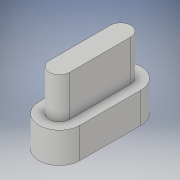
# Autodesk Inventor part: startselectButton
Saved by Autodesk Inventor 2019 (Build 230136000, 136)
## iProperties
Created: 2020-10-12
Part Number: startselectButton
Material: Generisch
Document SubType Name: Modeling
Designer: d_fel
Density: 1 g/cm^3
Appearance: Vorgabe
Author: d_fel
Autodesk Inventor part; units mm, degrees
ref_plane "YZ Plane" through (0, 0, 0) normal (1, 0, 0) x (0, 1, 0)
ref_plane "XZ Plane" through (0, 0, 0) normal (0, 1, 0) x (-1, 0, 0)
ref_plane "XY Plane" through (0, 0, 0) normal (0, 0, 1) x (1, 0, 0)
sketch "Skizze1" plane through (0, 0, 0) normal (0, 1, 0) x (-1, 0, 0)
  line L0 (4, 0) -> (4, -6)
  line L1 (0, -6) -> (0, 0)
  arc A0 (4, 0) -> (0, 0) centre (2, 0) ccw
  arc A1 (0, -6) -> (4, -6) centre (2, -6) ccw
  dimension "d0" = 4
  dimension "d1" = 6
  constraints: 4 end point, 4 point on circle, 4 tangent, 2 centre point, 1 parallel
  measures "d0" distance of L0.end L1.start
  measures "d1" distance of L0.start L0.end
extrude "Extrusion1" add sketch "Skizze1" along normal blind 3
sketch "Skizze2" plane through (0, 3, 0) normal (0, 1, 0) x (1, 0, 0)
  line L0 (-3, 0) -> (-3, 6)
  line L1 (-1, 6) -> (-1, 0)
  arc A0 (-3, 0) -> (-1, 0) centre (-2, 0) ccw
  arc A1 (-1, 6) -> (-3, 6) centre (-2, 6) ccw
  point P0 (0, 0)
  dimension "d4" = 2
  dimension "d5" = 6
  dimension "d6" = 1
  dimension "d7" = 0
  constraints: 4 end point, 4 point on circle, 4 tangent, 2 centre point, 1 horizontal alignment, 1 parallel
  measures "d4" distance between parallel lines of L0 L1
  measures "d5" distance of L0.start L0.end
  measures "d6" distance of point (0, 0) L1.end
  measures "d7" vertical distance of point (0, 0) L1.end
extrude "Extrusion2" add sketch "Skizze2" along normal blind 4
